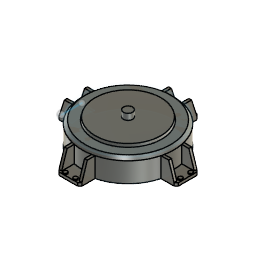
robotic_arm_base (Autodesk Fusion 360 design; units mm, degrees)
part number: 2026-02-28-09-25-21-614
Autodesk Fusion 360 part; units mm, degrees
sketch "Sketch1" plane through (0, 0, 0) normal (0, 0, 1) x (1, 0, 0)
  circle A0 centre (0, 0) radius 150
  dimension "d1" = 300
  constraint coincident A0.centre origin
  measures "d1" diameter of A0
extrude "Extrude1" add sketch "Sketch1" along normal blind 75
sketch "Sketch2" plane through (0, 0, 75) normal (0, 0, 1) x (-1, 0, 0)
  circle A0 centre (0, 0) radius 150
chamfer "Chamfer1" distance 10 angle 45 1 edges at (-139.8491, -54.2423, 75)
sketch "Sketch3" plane through (0, 0, 0) normal (0, 0, -1) x (1, 0, 0)
  circle A0 centre (0, 0) radius 150
  line L0 (0, 0) -> (-150, 0)
  line L1 (-195.2369, -37.5) -> (-145.2369, -37.5)
  line L2 (-145.2369, 37.5) -> (-195.2369, 37.5)
  line L3 (-195.2369, 37.5) -> (-195.2369, -37.5)
  line L4 (-195.2369, -37.5) -> (-150, 0) construction
  line L5 (-150, 0) -> (-195.2369, 37.5) construction
  circle A1 centre (0, 0) radius 150
  circle A2 centre (0, 0) radius 150
  point P0 (-150, 0)
  dimension "d5" = 50
  dimension "d6" = 50
  dimension "d7" = 75
  constraint coincident A0.centre L0.start
  constraint coincident A0 P0
  constraint horizontal L0
  constraint horizontal L1
  constraint parallel L1 L2
  constraint coincident L4 P0
  constraint coincident L5 P0
  constraint coincident P0 L0.end
  constraint coincident A0 L2.start
  constraint coincident A0 L1.end
  constraint symmetric L0 L1 L2
  measures "d5" distance of L2.end L2.start
  measures "d6" distance of L1.start L1.end
  measures "d7" distance of L1.start L2.end
extrude "Extrude2" add sketch "Sketch3" against normal blind 10 contours A0 L1 L2 L3 A1 A2
sketch "Sketch4" plane through (0, 0, 10) normal (0, 0, 1) x (-1, 0, 0)
  line L0 (195.2369, 37.5) -> (145.2369, 37.5)
  arc A0 (145.2369, -37.5) -> (145.2369, 37.5) centre (0, 0) ccw
  line L1 (145.2369, -37.5) -> (195.2369, -37.5)
  line L2 (195.2369, -37.5) -> (195.2369, 37.5)
sketch "Sketch5" plane through (0, 0, 0) normal (0, 0, -1) x (1, 0, 0)
  arc A0 (-145.2369, -37.5) -> (-145.2369, 37.5) centre (0, 0) ccw
  line L0 (-145.2369, 37.5) -> (-195.2369, 37.5)
  line L1 (-195.2369, 37.5) -> (-195.2369, -37.5)
  line L2 (-195.2369, -37.5) -> (-145.2369, -37.5)
chamfer "Chamfer2" distance 7 angle 45 1 edges at (-195.2369, -37.5, 5)
chamfer "Chamfer3" distance 7 angle 45 1 edges at (-195.2369, 37.5, 5)
sketch "Sketch6" plane through (0, 0, 0) normal (0, 0, -1) x (1, 0, 0)
sketch "Sketch7" plane through (0, 0, 0) normal (0, 0, -1) x (1, 0, 0)
sketch "Sketch8" plane through (0, 0, 0) normal (0, 0, -1) x (1, 0, 0)
sketch "Sketch9" plane through (0, 0, 0) normal (0, 0, -1) x (1, 0, 0)
sketch "Sketch10" plane through (0, -37.5, 0) normal (0, -1, 0) x (1, 0, 0)
  line L0 (-188.2369, 10) -> (-188.2369, 0)
  line L1 (-188.2369, 0) -> (-145.2369, 0)
  line L2 (-145.2369, 0) -> (-145.2369, 10)
  line L3 (-145.2369, 10) -> (-188.2369, 10)
  line L4 (-145.2369, 0) -> (-145.2369, 65)
  line L5 (-145.2369, 65) -> (-150, 65)
  line L6 (-150, 65) -> (-170.5569, 65)
  line L7 (-170.5569, 65) -> (-188.2369, 10)
  dimension "d12" = 17.68
  constraint coincident L1.end L2.start
  constraint perpendicular L1 L4
  constraint perpendicular L4 L5
  constraint perpendicular L4 L6
  constraint coincident L0.start L3.end
  measures "d12" horizontal distance of L6.end L0.start
extrude "Extrude3" add sketch "Sketch10" against normal blind 9 contours L3 L4 L5 L6 L7
sketch "Sketch11" plane through (0, 0, 10) normal (0, 0, 1) x (-1, 0, 0)
  line L0 (188.1828, 28.4628) -> (188.1828, -37.4441)
  constraint vertical L0
sketch "Sketch12" plane through (0, 0, 10) normal (0, 0, 1) x (-1, 0, 0)
  line L0 (182.2982, 13.1105) -> (188.2982, 9.6464)
  line L1 (188.2982, 9.6464) -> (194.2982, 13.1105)
  line L2 (194.2982, 13.1105) -> (194.2982, 20.0387)
  line L3 (194.2982, 20.0387) -> (188.2982, 23.5028)
  line L4 (188.2982, 23.5028) -> (182.2982, 20.0387)
  line L5 (182.2982, 20.0387) -> (182.2982, 13.1105)
  line L6 (188.2982, 16.5746) -> (188.2982, 9.6464)
  point P0 (188.2982, 16.5746)
  point P1 (188.1828, 28.4628)
  dimension "d15" = 6
  dimension "d16" = 4.96
  constraint coincident P0 L6.start
  measures "d15" distance of P0 L5
  measures "d16" vertical distance of L3.end P1
extrude "Extrude4" add sketch "Sketch12" along normal blind 3.5
ref_plane "WorkPlane1" through (-166.7369, 0, 32.5) normal (0, -1, 0) x (1, 0, 0)
mirror "Mirror1" about plane through (-166.7369, 0, 32.5) normal (0, -1, 0) of "Extrude3", "Extrude4"
pattern_circular "C-Pattern1" count 4 over 360 about axis through (0, 0, 1.75) along (0, 0, 1) of "Extrude2", "Chamfer2", "Chamfer3", "Extrude3", "Extrude4", "Mirror1"
sketch "Sketch13" plane through (0, 0, 75) normal (0, 0, 1) x (-1, 0, 0)
  circle A0 centre (0, 0) radius 110
  dimension "d23" = 220
  constraint coincident A0.centre origin
  measures "d23" diameter of A0
extrude "Extrude5" add sketch "Sketch13" along normal blind 9 draft -15
sketch "Sketch14" plane through (0, 0, 84) normal (0, 0, 1) x (-1, 0, 0)
  circle A0 centre (0, 0) radius 107.5885
  circle A1 centre (0, 0) radius 15
  dimension "d26" = 30
  constraint coincident A0.centre A1.centre
  measures "d26" diameter of A1
extrude "Extrude6" add sketch "Sketch14" along normal blind 20 contours A1
